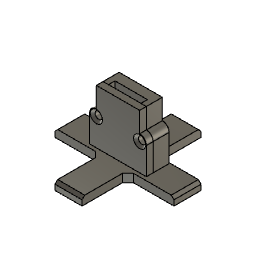
ピンセット台簡単 v2 (Autodesk Fusion 360 design; units mm, degrees)
Autodesk Fusion 360 part; units mm, degrees
note: some values were not read from the file. Chosen so that the rebuilt part matches the saved one: which bodies a step acts on; which face or edge a step refers to; which pieces of a blend or face edit are solid. Set by a fixed rule: which sketch regions a step uses.
sketch "スケッチ1" plane through (0, 0, 0) normal (0, 0, 1) x (1, 0, 0)
  line L0 (6.05, -1.2) -> (-6.05, -1.2)
  line L1 (-6.05, -1.2) -> (-6.05, 1.2)
  line L2 (-6.05, 1.2) -> (6.05, 1.2)
  line L3 (6.05, 1.2) -> (6.05, -1.2)
  line L4 (10, -6) -> (-10, -6)
  line L5 (-10, -6) -> (-10, 6)
  line L6 (-10, 6) -> (10, 6)
  line L7 (10, 6) -> (10, -6)
  dimension "d3" = 12.1
  dimension "d4" = 2.4
  dimension "d5" = 20
  dimension "d6" = 12
  constraint horizontal L0
  constraint perpendicular L0 L1
  constraint parallel L0 L2
  constraint parallel L1 L3
  constraint horizontal L4
  constraint perpendicular L4 L5
  constraint parallel L4 L6
  constraint parallel L5 L7
  measures "d3" distance of L1.end L2.end
  measures "d4" distance of L0.end L1.end
  measures "d5" distance of L5.end L6.end
  measures "d6" distance of L4.start L6.end
extrude "押し出し1" add sketch "スケッチ1" along normal blind 30 makes body 1
sketch "スケッチ2" plane through (0, 0, 0) normal (0, 0, 1) x (1, 0, 0)
  line L0 (20, -20) -> (-20, -20)
  line L1 (-20, -20) -> (-20, 20)
  line L2 (-20, 20) -> (20, 20)
  line L3 (20, 20) -> (20, -20)
  dimension "d9" = 40
  dimension "d10" = 40
  constraint horizontal L0
  constraint perpendicular L0 L1
  constraint parallel L0 L2
  constraint parallel L1 L3
  measures "d9" distance of L1.end L2.end
  measures "d10" distance of L0.end L1.end
extrude "押し出し2" add sketch "スケッチ2" along normal blind 5 separate body makes body 2
draft "勾配1" angle 15 neutral plane through (0, 0, 30) pull (0, 0, 1) 1 faces at (3.3333, -6, 10) on bodies 1
draft "勾配2" angle 15 neutral plane through (0, 0, 30) pull (0, 0, 1) 1 faces at (-3.3333, 6, 10) on bodies 1
draft "勾配3" angle 15 neutral plane through (0, 0, 30) pull (0, 0, 1) 1 faces at (10, 2, 10) on bodies 1
draft "勾配4" angle 15 neutral plane through (0, 0, 30) pull (0, 0, 1) 1 faces at (-10, -2, 10) on bodies 1
fillet "フィレット1" radius 1 4 edges at (0, 1.2, 30) (6.05, 0, 30) (0, -1.2, 30) (-6.05, 0, 30) on bodies 1
fillet "フィレット2" radius 0.5 4 edges at (-14.0192, 10.0192, 15) (14.0192, 10.0192, 15) (14.0192, -10.0192, 15) (-14.0192, -10.0192, 15) on bodies 1
fillet "フィレット3" radius 0.5 8 edges at (9.8604, -5.8604, 30) (10, 0, 30) (9.8604, 5.8604, 30) (0, 6, 30) (-9.8604, 5.8604, 30) (-10, 0, 30) (-9.8604, -5.8604, 30) (0, -6, 30) on bodies 1
fillet "フィレット4" radius 1 4 edges at (-20, 0, 5) (0, 20, 5) (20, 0, 5) (0, -20, 5) on bodies 2
sketch "スケッチ3" plane through (0, 0, 0) normal (0, 0, 1) x (1, 0, 0)
  line L0 (6, -1.3) -> (-6, -1.3)
  line L1 (-6, -1.3) -> (-6, 1.3)
  line L2 (-6, 1.3) -> (6, 1.3)
  line L3 (6, 1.3) -> (6, -1.3)
  line L4 (6, -1.3) -> (-6, 1.3) construction
  line L5 (-6, -1.3) -> (6, 1.3) construction
  line L6 (8, -3.3) -> (-8, -3.3)
  line L7 (-8, -3.3) -> (-8, 3.3)
  line L8 (-8, 3.3) -> (8, 3.3)
  line L9 (8, 3.3) -> (8, -3.3)
  line L10 (8, -3.3) -> (-8, 3.3) construction
  line L11 (-8, -3.3) -> (8, 3.3) construction
  dimension "d29" = 12
  dimension "d30" = 2.6
  dimension "d31" = 16
  dimension "d32" = 6.6
  constraint horizontal L0
  constraint perpendicular L0 L1
  constraint parallel L0 L2
  constraint parallel L1 L3
  constraint coincident L4 origin
  constraint coincident L5 origin
  constraint horizontal L6
  constraint perpendicular L6 L7
  constraint parallel L6 L8
  constraint parallel L7 L9
  constraint coincident L10 origin
  constraint coincident L11 origin
  measures "d29" distance of L1.end L2.end
  measures "d30" distance of L0.end L1.end
  measures "d31" distance of L7.end L8.end
  measures "d32" distance of L6.end L7.end
extrude "押し出し3" add sketch "スケッチ3" along normal blind 20 separate body makes body 3
sketch "スケッチ4" plane through (0, 0, 0) normal (0, 0, 1) x (1, 0, 0)
  line L0 (20, 5) -> (-20, 5)
  line L1 (-20, 5) -> (-20, -5)
  line L2 (-20, -5) -> (20, -5)
  line L3 (20, -5) -> (20, 5)
  line L4 (20, 5) -> (-20, -5) construction
  line L5 (-20, 5) -> (20, -5) construction
  line L6 (5, 20) -> (-5, 20)
  line L7 (-5, 20) -> (-5, -20)
  line L8 (-5, -20) -> (5, -20)
  line L9 (5, -20) -> (5, 20)
  line L10 (5, 20) -> (-5, -20) construction
  line L11 (-5, 20) -> (5, -20) construction
  dimension "d35" = 40
  dimension "d36" = 10
  dimension "d37" = 10
  dimension "d38" = 40
  constraint horizontal L0
  constraint perpendicular L0 L1
  constraint parallel L0 L2
  constraint parallel L1 L3
  constraint coincident L4 origin
  constraint coincident L5 origin
  constraint horizontal L6
  constraint perpendicular L6 L7
  constraint parallel L6 L8
  constraint parallel L7 L9
  constraint coincident L10 origin
  constraint coincident L11 origin
  measures "d35" distance of L1.end L2.end
  measures "d36" distance of L0.end L1.end
  measures "d37" distance of L7.end L8.end
  measures "d38" distance of L6.end L7.end
extrude "押し出し4" add sketch "スケッチ4" against normal blind 3 separate body makes body 4
split "分割1" by plane through (6, -1.3, 0) normal (0, -1, 0) bodies 3 makes body 5 at (-2.6667, 3.3, 13.3333)
sketch "スケッチ5" plane through (0, -3.3, 0) normal (0, -1, 0) x (1, 0, 0)
  line L0 (-8, 0) -> (8, 0)
  line L1 (8, 0) -> (8, 20)
  line L2 (8, 20) -> (-8, 20)
  line L3 (-8, 20) -> (-8, 0)
  line L4 (0, 20) -> (0, 0)
  circle A0 centre (-8, 10) radius 2.5
  circle A1 centre (-8, 10) radius 1.35
  circle A2 centre (-8, 10) radius 0.95
  dimension "d41" = 5
  dimension "d42" = 2.7
  dimension "d43" = 1.9
  constraint midpoint L2 L4.start
  constraint coincident L4.end origin
  constraint concentric A0 A1
  constraint concentric A0 A2
  measures "d41" diameter of A0
  measures "d42" diameter of A1
  measures "d43" diameter of A2
extrude "押し出し5" add sketch "スケッチ5" against normal blind 2 contours L3 A0 A1 | L3 A0 A1 bodies 3
extrude "押し出し6" cut sketch "スケッチ5" against normal blind 4 contours L3 A1 A2 | L3 A2 picked at (-7.4382, 11.0759) picked at (-7.5646, 10.0606) bodies 3
extrude "押し出し7" add sketch "スケッチ5" along normal blind -2 and the other way blind 6.6 contours L3 A0 A1 | L3 A1 A2 | L3 A1 A2 picked at (-8.1242, 7.8926) bodies 5
extrude "押し出し8" cut sketch "スケッチ5" against normal blind 11 contours L3 A2 | L3 A2 bodies 5
sketch "スケッチ6" plane through (0, 0, 0) normal (0, 0, -1) x (1, 0, 0)
  line L0 (8, 1.3) -> (6, 1.3)
  line L1 (6, 1.3) -> (6, -1.3)
  line L2 (6, -1.3) -> (-6, -1.3)
  line L3 (-6, -1.3) -> (-6, 1.3)
  line L4 (-6, 1.3) -> (-8, 1.3)
  line L5 (-8, 1.3) -> (-8, -3.3)
  line L6 (-8, -3.3) -> (8, -3.3)
  line L7 (8, -3.3) -> (8, 1.3)
  circle A0 centre (-8, -1) radius 2.3
  line L8 (-8, 1.3) -> (-10.5, 1.3)
  line L9 (-10.5, 1.3) -> (-10.5, -3.3)
  line L10 (-8, -3.3) -> (-8, 1.3)
  line L11 (-8, -3.3) -> (-10.5, -3.3)
  circle A1 centre (-8, -1) radius 1.35
  circle A2 centre (-8, -1) radius 0.95
  dimension "d54" = 2.7
  dimension "d55" = 1.9
  constraint midpoint L5 A0.centre
  constraint coincident L5.end A0
  constraint horizontal L8
  constraint vertical L9
  constraint vertical L10
  constraint coincident L4.end L5.start
  constraint coincident L5.end L6.start
  constraint tangent A0 L11
  constraint perpendicular L9 L11
  constraint concentric A0 A1
  constraint concentric A0 A2
  measures "d54" diameter of A1
  measures "d55" diameter of A2
extrude "押し出し9" add sketch "スケッチ6" against normal blind 10 contours L5 A0 L10 A1 | A0 L8 L9 L11 | L5 L10 A1 A2 picked at (-8.1143, 0.2081) bodies 5
delete_face "面を削除1" 1 faces at (-8.4059, 2.8372, 10) on bodies 5
extrude "押し出し10" cut sketch "スケッチ5" against normal blind 4.6 contours L3 A2 | L3 A2 bodies 5
delete_face "面を削除2" 1 faces at (-8.9397, 0.8607, 2.5612) on bodies 5
sketch "スケッチ7" plane through (0, 0, 0) normal (0, 0, -1) x (1, 0, 0)
extrude "押し出し11" cut sketch "スケッチ6" against normal blind 7.5 contours L5 L10 A2 | L5 L10 A2 bodies 5
split "分割2" by curves path "スケッチ5" along L4 bodies 5 makes body 6 at (-2.35, 3.3, 10)
delete_body "RemoveBody1" bodies 5
extrude "押し出し12" cut sketch "スケッチ6" along normal blind 4 contours L5 L10 A1 A2 | L5 L10 A1 A2 | L5 L10 A2 | L5 L10 A2 bodies 4
split "分割3" by plane through (0, 0, 0) normal (1, 0, 0) bodies 4 makes body 7 at (15, -1.6667, 0)
delete_body "RemoveBody2" bodies 7
split "分割4" by plane through (0, 0, 0) normal (1, 0, 0) bodies 3 makes body 8 at (2.6667, -3.3, 13.3333)
delete_body "RemoveBody3" bodies 8
chamfer "面取り1" distance 1 angle 45 1 edges at (-9.2586, 0.5118, -3) on bodies 4
sketch "スケッチ8" plane through (0, -1.3, 0) normal (0, -1, 0) x (1, 0, 0)
  circle A0 centre (-8, 10) radius 0.95
  line L0 (-10.5, 0) -> (-6, 0)
  line L1 (-6, 0) -> (-6, 20)
  line L2 (-6, 20) -> (-8, 20)
  line L3 (-8, 20) -> (-8, 12.5)
  arc A1 (-8, 12.5) -> (-10.5, 10) centre (-8, 10) ccw
  line L4 (-10.5, 10) -> (-10.5, 0)
extrude "押し出し13" add sketch "スケッチ8" along normal blind 2 bodies 3 4
extrude "押し出し14" cut sketch "スケッチ5" against normal blind 5 contours L3 A1 A2 | L3 A1 A2 bodies 3
move_face "面を移動1" by (0, -0.1, 0) 1 faces at (-4, 1.3, 13.3333) on bodies 6
move_face "面を移動2" by (0, 0.1, 0) 1 faces at (-2.2167, -1.3, 10) on bodies 3
move_face "面を移動3" by (0, 0.1, 0) 1 faces at (-8.1903, -1.3, 3.0176) on bodies 6
chamfer "面取り2" distance 2 angle 45 2 edges at (-5, 5, -1.5) (-5, -5, -1.5) on bodies 3
move_face "面を移動4" by (0, 2, 0) 1 faces at (-1.6667, 20, -1) on bodies 3
move_face "面を移動5" by (0, -2, 0) 1 faces at (-3.3333, -20, -1) on bodies 3
move_face "面を移動6" by (-2, 0, 0) 1 faces at (-20, 1.6667, -1) on bodies 3
split "分割5" by plane through (0, 20, 0) normal (0, 0, 1) bodies 3 makes body 9 at (-2.2167, -3.3, 10)
chamfer "面取り3" distance 1 angle 45 1 edges at (-22, 0, 0) on bodies 3
chamfer "面取り4" distance 1 angle 45 1 edges at (-2.5, 22, 0) on bodies 3
chamfer "面取り5" distance 1 angle 45 1 edges at (-2.5, -22, 0) on bodies 3
mirror "ミラー1" about plane through (0, 20, 0) normal (1, 0, 0) of bodies 3 merged
mirror "ミラー2" about plane through (0, 996.7, 20) normal (1, 0, 0) of bodies 6 merged
chamfer "面取り6" distance 0.9 angle 45 1 edges at (-9.2586, -3.3, 10.4882) on bodies 9
mirror "ミラー3" about plane through (0, 20, 0) normal (1, 0, 0) of bodies 9 makes body 10
combine "結合1" operation add target body 9 tool bodies 10
move_face "面を移動7" by (0, 1.4, 0) 1 faces at (2.4345, 3.3, 3.1179) on bodies 6
move_body "移動1" bodies 9 to x (1, 0, 0) y (0, 1, 0) z (0, 0, 1) at (0, -0.4, 0)
move_face "面を移動8" by (0, 0.4, 0) 1 faces at (2.3861, -1.6, 2.9815) on bodies 9
hidden bodies 1 2
named bodies: "01", "02", "03", "03 (1)"
